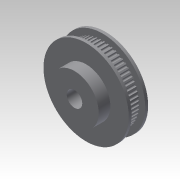
# Autodesk Inventor part: GT2 60T Drive Pulley
Saved by Autodesk Inventor 2020 (Build 240168000, 168)
## iProperties
Created: 2015-06-17
Part Number: GT2 60T Drive Pulley
Material: Generic
Document SubType Name: Modeling
Designer: Andrew
Density: 1 g/cm^3
Appearance: Default
Author: Andrew
Autodesk Inventor part; units mm, degrees
ref_plane "YZ Plane" through (0, 0, 0) normal (1, 0, 0) x (0, 1, 0)
ref_plane "XZ Plane" through (0, 0, 0) normal (0, 1, 0) x (-1, 0, 0)
ref_plane "XY Plane" through (0, 0, 0) normal (0, 0, 1) x (1, 0, 0)
sketch "Sketch1" plane through (0, 0, 0) normal (0, 0, 1) x (1, 0, 0)
  line L0 (0, 0) -> (0, 16) construction
  line L1 (0, 16) -> (4, 16) construction
  line L2 (4, 16) -> (22, 16)
  line L3 (22, 16) -> (22, 14.5)
  line L4 (22, 14.5) -> (18.95, 14.5)
  line L5 (18.95, 14.5) -> (18.95, 7.5)
  line L6 (18.95, 7.5) -> (22, 7.5)
  line L7 (4, 0) -> (4, 16)
  line L8 (4, 0) -> (12.5, 0)
  line L9 (12.5, 0) -> (12.5, 6)
  line L10 (12.5, 6) -> (22, 6)
  line L11 (22, 6) -> (22, 7.5)
  dimension "d0" = 4
  dimension "d1" = 7
  dimension "d4" = 1.5
  dimension "d6" = 18.95
  dimension "d15" = 22
  dimension "d16" = 6
  dimension "d17" = 12.5
  constraints: 24 end point, 8 perpendicular, 3 point on line, 1 collinear, 1 horizontal, 1 parallel, 1 vertical
  measures "d0" distance between parallel lines of L0 L7
  measures "d1" distance of L4.end L5.end
  measures "d4" distance between parallel lines of L2 L4
  measures "d6" distance between parallel lines of L0 L5
  measures "d15" distance between parallel lines of L0 L3
  measures "d16" distance of L8.end L9.end
  measures "d17" distance between parallel lines of L0 L9
revolve "Revolution1" add sketch "Sketch1" angle 360 about axis through (0, 0, 0) along (0, 1, 0)
sketch "Sketch2" plane through (0, 7.5, 0) normal (0, 1, 0) x (1, 0, 0)
  line L0 (0, 0) -> (0, -18.85)
  circle A0 centre (0, -18.85) radius 0.65
  dimension "d8" = 1.3
  dimension "d9" = 18.85
  constraints: 2 end point, 1 centre point, 1 coincident, 1 vertical
  measures "d8" diameter of A0
  measures "d9" distance of L0.start L0.end
extrude "Extrusion1" cut sketch "Sketch2" along normal up to surface (7 mm away)
pattern_circular "Circular Pattern1" count 60 over 360 about axis through (0, 11, 0) along (0, -1, 0) of "Extrusion1"
body "Solid1"
